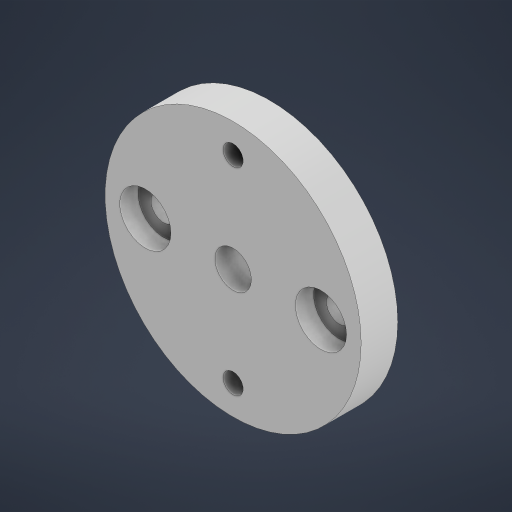
# Autodesk Inventor part: Crank
Saved by Autodesk Inventor 2024 (Build 280153000, 153)
## iProperties
Created: 2023-12-06
Part Number: Crank
Material: Generic
Document SubType Name: Modeling
Designer: calvi
Density: 1 g/cm^3
Appearance: Default
Author: calvi
Autodesk Inventor part; units mm, degrees
ref_plane "YZ Plane" through (0, 0, 0) normal (1, 0, 0) x (0, 1, 0)
ref_plane "XZ Plane" through (0, 0, 0) normal (0, 1, 0) x (-1, 0, 0)
ref_plane "XY Plane" through (0, 0, 0) normal (0, 0, 1) x (1, 0, 0)
sketch "Sketch1" plane through (0, 0, 0) normal (0, 0, 1) x (1, 0, 0)
  circle A0 centre (0, 0) radius 44.45
  dimension "d0" = 88.9
  constraints: 1 centre point, 1 coincident
  measures "d0" diameter of A0
extrude "Extrusion1" add sketch "Sketch1" along normal blind 19.05
sketch "Sketch2" plane through (0, 0, 19.05) normal (0, 0, 1) x (1, 0, 0)
  circle A0 centre (0, 34.29) radius 3.4925
  circle A1 centre (0, -34.29) radius 3.4925
  point P0 (0, 0)
  dimension "d3" = 6.985
  dimension "d4" = 34.29
  dimension "d5" = 6.985
  dimension "d6" = 34.29
  constraints: 2 centre point, 2 vertical alignment
  measures "d3" diameter of A0
  measures "d4" distance of point (0, 0) A0.centre
  measures "d5" diameter of A1
  measures "d6" distance of point (0, 0) A1.centre
sketch "Sketch3" plane through (0, 0, 19.05) normal (0, 0, 1) x (1, 0, 0)
  circle A0 centre (0, 0) radius 44.45
  dimension "d9" = 88.9
  constraints: 1 centre point, 1 coincident
  measures "d9" diameter of A0
extrude "Extrusion3" cut sketch "Sketch3" against normal blind 6.35
sketch "Sketch4" plane through (0, 0, 12.7) normal (0, 0, 1) x (1, 0, 0)
  circle A0 centre (0, 0) radius 6.35
  dimension "d12" = 12.7
  constraints: 1 centre point, 1 coincident
  measures "d12" diameter of A0
extrude "Extrusion4" cut sketch "Sketch2" against normal blind 26.9875
extrude "Extrusion5" cut sketch "Sketch4" against normal blind 44.45
sketch "Sketch5" plane through (0, 0, 12.7) normal (0, 0, 1) x (1, 0, 0)
  circle A0 centre (-30.48, 0) radius 4.445
  circle A1 centre (0, 0) radius 6.35 projected
  circle A2 centre (0, 34.29) radius 3.4925 projected
  line L0 (0, 0) -> (0, 34.29)
  circle A3 centre (30.48, 0) radius 4.445
  dimension "d17" = 8.89
  dimension "d18" = 30.48
  dimension "d19" = 34.29
  constraints: 2 centre point, 2 end point, 1 symmetric about line, 1 vertical, 1 other
  measures "d17" diameter of A0
  measures "d18" distance of L0.start A0.centre
  measures "d19" vertical distance of L0.end A0.centre
extrude "Extrusion6" cut sketch "Sketch5" against normal blind 80.9625 contours A0 | A3
sketch "Sketch6" plane through (0, 0, 12.7) normal (0, 0, 1) x (1, 0, 0)
  circle A0 centre (-30.48, 0) radius 8.89
  circle A1 centre (0, 34.29) radius 3.4925 projected
  line L0 (0, 0) -> (0, 34.29)
  circle A2 centre (30.48, 0) radius 8.89
  circle A3 centre (-30.48, 0) radius 4.445
  circle A4 centre (-30.48, 0) radius 4.445 projected
  circle A5 centre (30.48, 0) radius 4.445
  dimension "d22" = 17.78
  dimension "d23" = 30.48
  dimension "d24" = 34.29
  dimension "d25" = 0
  constraints: 4 centre point, 2 end point, 2 symmetric about line, 1 coincident, 1 vertical, 2 other
  measures "d22" diameter of A0
  measures "d23" distance of L0.start A0.centre
  measures "d24" vertical distance of A0.centre L0.end
  measures "d25" radial gap between concentric circles of A4 A3
extrude "Extrusion7" cut sketch "Sketch6" against normal blind 6.35 contours A0 | A2
sketch "Sketch8" plane through (-30.48, 0, 6.35) normal (0, 0, 1) x (1, 0, 0)
  circle A0 centre (0, 0) radius 4.445
  circle A1 centre (0, 0) radius 8.89
  circle A2 centre (0, 0) radius 4.445 projected
  circle A3 centre (0, 0) radius 8.89 projected
  circle A4 centre (30.48, 34.29) radius 3.4925 projected
  line L0 (30.48, 34.29) -> (30.48, 0)
  circle A5 centre (60.96, 0) radius 4.445
  circle A6 centre (60.96, 0) radius 8.89
  dimension "d28" = 0
  dimension "d29" = 0
  dimension "d30" = 30.48
  dimension "d31" = 34.29
  constraints: 4 centre point, 2 coincident, 2 end point, 2 symmetric about line, 1 vertical, 2 other
  measures "d28" radial gap between concentric circles of A0 A2
  measures "d29" radial gap between concentric circles of A1 A3
  measures "d30" distance of L0.end A0.centre
  measures "d31" vertical distance of A0.centre L0.start
extrude "Extrusion8" add sketch "Sketch8" against normal blind 9.525 contours A1 | A6
body "Solid1"
